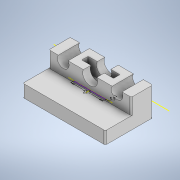
# Autodesk Inventor part: QuickDisconnetPrintHeadMount
Saved by Autodesk Inventor 2021 (Build 250183000, 183)
## iProperties
Created: 2021-11-11
Part Number: QuickDisconnetPrintHeadMount
Material: Generic
Document SubType Name: Sheet Metal
Designer: Unit-005
Density: 1 g/cm^3
Sheet Metal Rule: Default
Appearance: Default
Author: Unit-005
## iProperties of the stored document _3DPrint.ipt
Created: 2021-11-11
Part Number: _3DPrint
Material: Generic
Document SubType Name: Modeling
Designer: Unit-005
Density: 1 g/cm^3
Appearance: Default
Author: Unit-005
Autodesk Inventor part; units mm, degrees
ref_plane "YZ Plane" through (0, 0, 0) normal (1, 0, 0) x (0, 1, 0)
ref_plane "XZ Plane" through (0, 0, 0) normal (0, 1, 0) x (-1, 0, 0)
ref_plane "XY Plane" through (0, 0, 0) normal (0, 0, 1) x (1, 0, 0)
sketch "Sketch1" plane through (0, 0, 0) normal (0, 0, 1) x (1, 0, 0)
  line L0 (-29, 10) -> (29, 10)
  line L1 (29, 10) -> (29, -10)
  line L2 (29, -10) -> (-29, -10)
  line L3 (-29, -10) -> (-29, 10)
  line L4 (-29, 10) -> (29, -10) construction
  line L5 (29, 10) -> (-29, -10) construction
  point P0 (0, 0)
  dimension "d0" = 58
  dimension "d1" = 20
  constraints: 12 end point, 2 midpoint, 2 parallel, 1 horizontal, 1 perpendicular
  measures "d0" distance of L1.end L2.end
  measures "d1" distance of L0.end L1.end
extrude "Extrusion1" add sketch "Sketch1" along normal blind 15
sketch "Sketch3" plane through (0, 0, 0) normal (0, 0, 1) x (1, 0, 0)
  line L0 (-29, -10) -> (29, -10) projected
  line L1 (29, -10) -> (29, 10) projected
  line L2 (29, 10) -> (-29, 10) projected
  line L3 (-29, 10) -> (-29, -10) projected
  line L4 (-40.6, 0) -> (40.6, 0) projected
  line L5 (0, -12.225) -> (0, 13.85) projected
  circle A0 centre (18.95, 7.75) radius 4.125
  circle A1 centre (-18.95, 7.75) radius 4.125
  point P0 (0, 0)
  point P1 (-22.4073, 10)
  point P2 (-15.4927, 10)
  point P3 (15.4927, 10)
  point P4 (22.4073, 10)
  dimension "d4" = 8.25
  dimension "d5" = 8.25
  dimension "d6" = 37.9
  dimension "d7" = 2.25
  constraints: 2 centre point, 1 symmetric about line
  measures "d4" diameter of A0
  measures "d5" diameter of A1
  measures "d6" distance of A1.centre A0.centre
  measures "d7" distance from line of L2 A0.centre
extrude "Extrusion2" cut sketch "Sketch3" along normal through all contours L2 A1 | L2 A0 picked at (-19.324, 7.5879) picked at (18.8469, 7.6595)
sketch "Sketch4" plane through (-15.4927, 10, 0) normal (0, 1, 0) x (1, 0, 0)
  line L0 (0, 0) -> (0, -15) projected
  line L1 (30.9853, -15) -> (0, -15) projected
  line L2 (30.9853, -15) -> (30.9853, 0) projected
  line L3 (30.9853, 0) -> (0, 0) projected
  line L4 (-25.1073, 0) -> (56.0927, 0) projected
  line L5 (15.4927, 0) -> (15.4927, -15) construction
  line L6 (30.9853, -15) -> (0, -15) construction
  line L7 (30.9853, -15) -> (30.9853, 0) construction
  line L8 (30.9853, -7.5) -> (0, -7.5) construction
  line L9 (4.2927, -5.25) -> (26.6927, -5.25)
  line L10 (26.6927, -5.25) -> (26.6927, -9.75)
  line L11 (26.6927, -9.75) -> (4.2927, -9.75)
  line L12 (4.2927, -9.75) -> (4.2927, -5.25)
  line L13 (4.2927, -5.25) -> (26.6927, -9.75)
  line L14 (26.6927, -5.25) -> (4.2927, -9.75)
  point P0 (15.4927, -7.5)
  dimension "d12" = 22.4
  dimension "d13" = 4.5
  constraints: 16 end point, 6 midpoint, 2 parallel, 1 horizontal, 1 perpendicular
  measures "d12" distance of L10.end L11.end
  measures "d13" distance of L9.end L10.end
sketch "Sketch5" plane through (0, 0, 0) normal (0, 1, 0) x (-1, 0, 0)
  line L0 (15.4927, 0) -> (15.4927, 15) projected
  line L1 (-15.4927, 15) -> (15.4927, 15) projected
  line L2 (-15.4927, 15) -> (-15.4927, 0) projected
  line L3 (-15.4927, 0) -> (15.4927, 0) projected
  line L4 (40.6, 0) -> (-40.6, 0) projected
  line L5 (0, -3.05) -> (0, 18.3) projected
  line L6 (11.25, 9.75) -> (-11.25, 9.75)
  line L7 (-11.25, 9.75) -> (-11.25, 15.25)
  line L8 (-11.25, 15.25) -> (11.25, 15.25)
  line L9 (11.25, 15.25) -> (11.25, 9.75)
  line L10 (11.25, 9.75) -> (-11.25, 15.25) construction
  line L11 (-11.25, 9.75) -> (11.25, 15.25) construction
  point P0 (0, 0)
  point P1 (0, 12.5)
  dimension "d10" = 22.5
  dimension "d11" = 5.5
  constraints: 12 end point, 2 midpoint, 2 parallel, 1 horizontal, 1 perpendicular, 1 point on line
  measures "d10" distance of L7.end L8.end
  measures "d11" distance of L6.end L7.end
extrude "Extrusion3" cut sketch "Sketch4" against normal blind 10 contours L13 L14 L12 | L9 L14 L13 | L10 L13 L14 | L14 L13 L11
sketch "Sketch6" plane through (0, 0, 0) normal (0, 0, -1) x (-1, 0, 0)
  line L0 (11.2, 0) -> (-11.2, 0) projected
  arc A0 (15.4927, 10) -> (22.4073, 10) centre (18.95, 7.75) ccw projected
  line L1 (-15.4927, 10) -> (15.4927, 10) projected
  arc A1 (-22.4073, 10) -> (-15.4927, 10) centre (-18.95, 7.75) ccw projected
  line L2 (-29, 10) -> (-22.4073, 10) projected
  line L3 (-29, -10) -> (-29, 10) projected
  line L4 (29, -10) -> (-29, -10) projected
  line L5 (29, 10) -> (29, -10) projected
  line L6 (22.4073, 10) -> (29, 10) projected
  line L7 (40.6, 0) -> (-40.6, 0) projected
  line L8 (0, -14.25) -> (0, 15.5) projected
  circle A2 centre (0, 7.75) radius 5.25
  point P0 (0, 0)
  dimension "d16" = 10.5
  constraints: 1 centre point, 1 horizontal alignment, 1 point on line
  measures "d16" diameter of A2
extrude "Extrusion4" cut sketch "Sketch6" against normal through all contours A2 L1 L8 | L8 L1 A2 | L8 A2 L1 | L1 A2 L8
sketch "Sketch8" plane through (0, 0, 15) normal (0, 0, 1) x (1, 0, 0)
  arc A0 (-4.7434, 10) -> (4.7434, 10) centre (0, 7.75) ccw projected
  line L0 (-4.7434, 10) -> (-15.4927, 10) projected
  arc A1 (-22.4073, 10) -> (-15.4927, 10) centre (-18.95, 7.75) ccw projected
  line L1 (-22.4073, 10) -> (-29, 10) projected
  line L2 (-29, 10) -> (-29, -10) projected
  line L3 (-29, -10) -> (29, -10) projected
  line L4 (29, -10) -> (29, 10) projected
  line L5 (29, 10) -> (22.4073, 10) projected
  arc A2 (15.4927, 10) -> (22.4073, 10) centre (18.95, 7.75) ccw projected
  line L6 (15.4927, 10) -> (4.7434, 10) projected
  line L7 (-40.6, 0) -> (40.6, 0) projected
  line L8 (0, -14) -> (0, 14) projected
  line L9 (-29, 10) -> (-29, -10) projected
  line L10 (29, -10) -> (-29, -10)
  line L11 (-29, -10) -> (-29, -1.25)
  line L12 (-29, -1.25) -> (29, -1.25)
  line L13 (29, -1.25) -> (29, -10)
  point P0 (0, 0)
  point P1 (29, -1.25)
  dimension "d19" = 9
  constraints: 8 end point, 2 parallel, 1 horizontal, 1 perpendicular, 1 point on line
  measures "d19" distance from line of A1.centre L12
extrude "Extrusion5" add sketch "Sketch8" along normal blind 18.3 contours L12 L4 L3 L8 | L8 L3 L2 L12
fillet "Fillet4" radius 1 4 edges at (-29, -5.625, 33.3) (29, -5.625, 33.3) (-29, 4.375, 15) (29, 4.375, 15)
fillet "Fillet5" radius 1 2 edges at (-29, 0, 0) (29, 0, 0)
fillet "Fillet6" radius 0.5 4 edges at (-11.2, 5, 5.25) (-11.2, 5, 9.75) (11.2, 5, 5.25) (11.2, 5, 9.75)
equation "\"BendRadius\" = Thickness"
equation "\"BendReliefWidth\" = Thickness"
equation "\"BendReliefDepth\" = 0.5 * Thickness"
equation "\"CornerReliefSize\" = 4 * Thickness"
equation "\"MinimumRemnant\" = 2 * Thickness"
equation "\"TransitionRadius\" = BendRadius"
equation "\"JacobiRadiusSize\" = BendRadius"
equation "\"GapSize\" = Thickness"
equation "\"Thickness\" = 3.048"
body "Solid1"
